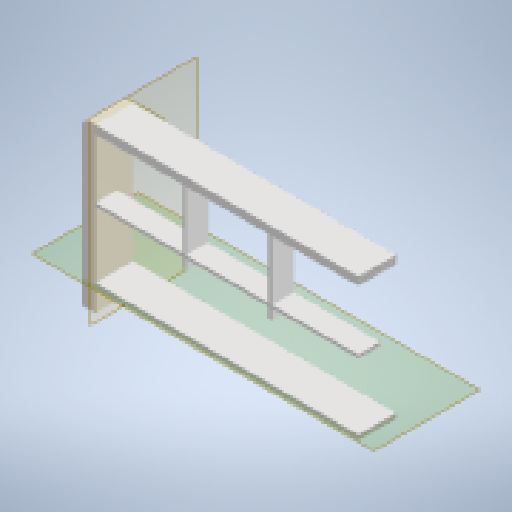
# Autodesk Inventor part: case
Saved by Autodesk Inventor 2024.3 (Build 283343000, 343)
## iProperties
Created: 2025-06-10
Part Number: case
Material: Generic
Document SubType Name: Modeling
Designer: megha
Density: 1 g/cm^3
Appearance: Default
Author: megha
Autodesk Inventor part; units mm, degrees
ref_plane "YZ Plane" through (0, 0, 0) normal (1, 0, 0) x (0, 1, 0)
ref_plane "XZ Plane" through (0, 0, 0) normal (0, 1, 0) x (-1, 0, 0)
ref_plane "XY Plane" through (0, 0, 0) normal (0, 0, 1) x (1, 0, 0)
ref_plane "boardTop(tolerance)" through (29.1257, 19.6924, 40.7272) normal (0, -1, 0) x (1, 0, 0)
sketch "Sketch3" plane through (29.1257, 19.6924, 40.7272) normal (0, -1, 0) x (1, 0, 0)
  line L0 (-2, 1.51) -> (-2, 0)
  line L1 (158.35, 0) -> (158.35, 1.51)
  line L2 (-11, 18.0177) -> (-11, -5)
  line L3 (167.35, 18.0177) -> (167.35, -5)
  line L4 (167.35, 18.0177) -> (-11, 18.0177)
  line L5 (-11, -5) -> (167.35, -5)
  point P0 (-29.1257, -40.7272)
  point P1 (158.35, 0.755)
  dimension "d12" = 9
  dimension "d13" = 9
  constraints: 12 end point, 1 horizontal, 1 midpoint, 1 parallel, 1 vertical, 2 other
  measures "d12" distance between parallel lines of L2 L0
  measures "d13" distance from line of point (158.35, 0.755) L3
extrude "Extrusion3" add sketch "Sketch3" against normal blind 5
ref_plane "boardBottom(tolerance)" through (185.4757, -59.8376, 42.2372) normal (0, -1, 0) x (-1, 0, 0)
sketch "Sketch4" plane through (29.1257, 19.6924, 40.7272) normal (0, -1, 0) x (1, 0, 0)
  line L0 (-2, 1.51) -> (-2, 0)
  line L1 (158.35, 1.51) -> (158.35, 0)
  line L2 (-11, 18.0177) -> (-11, -5) projected
  line L3 (-11, -5) -> (167.35, -5) projected
  line L4 (167.35, -5) -> (167.35, 18.0177) projected
  line L5 (167.35, 18.0177) -> (-11, 18.0177) projected
  line L6 (159.35, -5) -> (159.35, 18.0177)
  line L7 (-11, 18.0177) -> (167.35, 18.0177) projected
  line L8 (-3, -5) -> (-3, 18.0177)
  point P0 (-29.1257, -40.7272)
  point P1 (158.35, 0.755)
  point P2 (-2, 0.755)
  point P3 (-3, 18.0177)
  dimension "d17" = 1
  dimension "d18" = 1
  constraints: 8 end point, 4 point on line, 2 midpoint, 2 perpendicular, 2 vertical, 4 other
  measures "d17" distance from line of point (158.35, 0.755) L6
  measures "d18" distance from line of point (-2, 0.755) L8
extrude "Extrusion4" add sketch "Sketch4" along normal blind 94.5274 contours L5 L8 L3 L2 | L5 L4 L3 L6
ref_plane "boardRight(tolerance)" through (188.4757, 19.6924, 35.7272) normal (-1, 0, 0) x (0, -1, 0)
sketch "Sketch5" plane through (188.4757, -74.835, 35.7272) normal (-1, 0, 0) x (0, 0, 1)
  line L0 (5, 15.9974) -> (6.51, 15.9974) projected
  line L1 (0, 94.5274) -> (23.0177, 94.5274) projected
  line L2 (0, 94.5274) -> (0, 0) projected
  line L3 (23.0177, 0) -> (0, 0) projected
  line L4 (23.0177, 94.5274) -> (23.0177, 0) projected
  line L5 (0, 94.5274) -> (0, 0) projected
  line L6 (0, 15.9974) -> (23.0177, 15.9974)
  line L7 (23.0177, 15.9974) -> (23.0177, 12.9974)
  line L8 (23.0177, 12.9974) -> (0, 12.9974)
  line L9 (0, 12.9974) -> (0, 15.9974)
  point P0 (-35.7272, 74.835)
  point P1 (0, 12.9974)
  point P2 (6.51, 15.9974)
  dimension "d21" = 3
  constraints: 8 end point, 2 horizontal, 2 parallel, 2 point on line, 1 perpendicular
  measures "d21" distance of L6.end L7.end
ref_plane "boardLeft(tolerance)" through (26.1257, 19.6924, 58.7449) normal (1, 0, 0) x (0, -1, 0)
extrude "Extrusion5" add sketch "Sketch5" along normal up to surface (162.35 mm away) contours L0 L6 L4 L8 L2
sketch "Sketch6" plane through (29.1257, 19.6924, 40.7272) normal (0, -1, 0) x (1, 0, 0)
  line L0 (48.3131, 6.295) -> (48.54, 4.395) projected
  line L1 (54.3069, 2.495) -> (54.08, 4.395) projected
  line L2 (99.8531, 6.295) -> (100.08, 4.395) projected
  line L3 (107.5969, 2.495) -> (107.37, 4.395) projected
  line L4 (-3, 18.0177) -> (-3, -5) projected
  line L5 (-3, -5) -> (159.35, -5) projected
  line L6 (159.35, -5) -> (159.35, 18.0177) projected
  line L7 (159.35, 18.0177) -> (-3, 18.0177) projected
  line L8 (0, 1.51) -> (156.35, 1.51) projected
  line L9 (102.725, 1.51) -> (104.725, 1.51)
  line L10 (104.725, 1.51) -> (104.725, 18.0177)
  line L11 (104.725, 18.0177) -> (102.725, 18.0177)
  line L12 (102.725, 18.0177) -> (102.725, 1.51)
  line L13 (159.35, 18.0177) -> (-3, 18.0177) projected
  line L14 (50.31, 1.51) -> (52.31, 1.51)
  line L15 (52.31, 1.51) -> (52.31, 18.0177)
  line L16 (52.31, 18.0177) -> (50.31, 18.0177)
  line L17 (50.31, 18.0177) -> (50.31, 1.51)
  line L18 (48.4266, 5.345) -> (50.31, 5.345) construction
  line L19 (54.1934, 3.445) -> (52.31, 3.445) construction
  line L20 (99.9666, 5.345) -> (102.725, 5.345) construction
  line L21 (107.4834, 3.445) -> (104.725, 3.445) construction
  point P0 (-29.1257, -40.7272)
  point P1 (124.6421, 15.795)
  dimension "d31" = 2
  dimension "d32" = 2
  constraints: 24 end point, 8 point on line, 6 parallel, 6 perpendicular, 4 midpoint, 2 horizontal, 1 other
  measures "d31" distance between parallel lines of L17 L15
  measures "d32" distance between parallel lines of L10 L12
extrude "Extrusion6" add sketch "Sketch6" along normal blind 44.45 contours L7 L15 L8 L17 | L7 L10 L8 L12
sketch "Sketch7" plane through (133.8507, 19.6924, 42.2372) normal (0, 0, -1) x (-1, 0, 0)
  line L0 (2, 0) -> (2, -44.45) projected
  line L1 (0, 0) -> (0, -44.45) projected
  line L2 (2, -44.45) -> (0, -44.45) projected
  line L3 (54.415, 0) -> (54.415, -44.45) projected
  line L4 (52.415, 0) -> (52.415, -44.45) projected
  line L5 (54.415, -44.45) -> (52.415, -44.45) projected
  line L6 (0, 0) -> (2, 0)
  line L7 (54.415, 0) -> (52.415, 0)
  point P0 (133.8507, -19.6924)
  constraints: 4 end point, 1 collinear, 1 horizontal
extrude "Extrusion7" cut sketch "Sketch7" against normal blind 3
sketch "Sketch9" plane through (188.4757, 19.6924, 35.7272) normal (-1, 0, 0) x (0, 0, 1)
  line L0 (9.51, -38.275) -> (23.0177, -38.275)
  line L1 (9.51, -36.275) -> (23.0177, -36.275)
  line L2 (9.51, -36.275) -> (23.0177, -36.275)
  line L3 (23.0177, -36.275) -> (23.0177, -38.275)
  line L4 (23.0177, -38.275) -> (9.51, -38.275)
  line L5 (9.51, -38.275) -> (9.51, -36.275)
  point P0 (-35.7272, -19.6924)
  dimension "d37" = 2
  constraints: 12 end point, 3 horizontal, 2 parallel, 1 perpendicular
  measures "d37" distance between parallel lines of L0 L1
extrude "Extrusion8" add sketch "Sketch9" along normal up to surface (162.35 mm away)
fillet "Fillet1" radius 4.7625 2 edges at (18.1257, 24.6924, 47.236) (196.4757, 24.6924, 47.236)
sketch "Sketch10" plane through (196.4757, 19.6924, 35.7272) normal (-1, 0, 0) x (0, 0, 1)
  line L0 (10.3897, -67.2551) -> (10.3897, -61.4051) projected
  line L1 (7.715, -63.9401) -> (7.715, -66.58) projected
  line L2 (9.495, -60.3354) -> (8.9571, -60.3354) projected
  line L3 (8.9571, -68.3248) -> (9.495, -68.3248) projected
  arc A0 (10.145, -61.0301) -> (9.695, -60.5801) centre (9.695, -61.0301) ccw projected
  line L4 (8.4889, -60.7119) -> (7.8268, -61.374) projected
  line L5 (7.8268, -67.2862) -> (8.4889, -67.9483) projected
  line L6 (7.715, -62.0803) -> (7.715, -63.9301) projected
  line L7 (7.715, -63.9401) -> (7.715, -66.58) projected
  line L8 (10.3897, -67.2551) -> (10.3897, -61.4051) projected
  line L9 (11.2274, -71.6801) -> (6.8774, -71.6801)
  line L10 (4.8774, -69.6801) -> (4.8774, -58.9801)
  line L11 (6.8774, -56.9801) -> (11.2274, -56.9801)
  line L12 (13.2274, -58.9801) -> (13.2274, -69.6801)
  line L13 (9.226, -68.3248) -> (9.2261, -71.6801) construction
  line L14 (9.226, -60.3354) -> (9.226, -56.9801) construction
  line L15 (13.2274, -64.3301) -> (10.3897, -64.3301) construction
  line L16 (7.715, -64.3301) -> (4.8774, -64.3301) construction
  arc A1 (13.2274, -58.9801) -> (11.2274, -56.9801) centre (11.2274, -58.9801) ccw
  arc A2 (6.8774, -56.9801) -> (4.8774, -58.9801) centre (6.8774, -58.9801) ccw
  arc A3 (4.8774, -69.6801) -> (6.8774, -71.6801) centre (6.8774, -69.6801) ccw
  arc A4 (11.2274, -71.6801) -> (13.2274, -69.6801) centre (11.2274, -69.6801) ccw
  point P0 (-35.7272, -19.6924)
  point P1 (7.685, -61.1849)
  point P2 (13.2274, -71.6801)
  point P3 (4.8774, -56.9801)
  point P4 (4.8774, -71.6801)
  point P5 (13.2274, -56.9801)
  point P6 (9.495, -68.3248)
  dimension "d47" = 8.35
  dimension "d48" = 14.7
  dimension "d49" = 2
  constraints: 16 end point, 13 point on line, 8 point on circle, 8 tangent, 5 midpoint, 4 centre point, 3 equal radius, 2 collinear, 2 parallel, 2 perpendicular, 1 horizontal, 2 other
  measures "d47" distance of point (4.877, -56.98) point (13.227, -56.98)
  measures "d48" distance of point (13.227, -56.98) point (13.227, -71.68)
  measures "d49" radius of A1
extrude "Extrusion9" cut sketch "Sketch10" along normal blind 8
body "Solid2"
